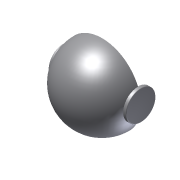
# Autodesk Inventor part: Head
Saved by Autodesk Inventor 2011 (Build 150239000, 239)
## iProperties
Created: 2011-04-09
Part Number: Head
Document SubType Name: Modeling
Designer: Milton
Density: 1 g/cm^3
Author: Milton
Autodesk Inventor part; units mm, degrees
sketch "Sketch1" plane through (0, 0, 0) normal (0, 0, 1) x (1, 0, 0)
  arc A0 (-59, 0) -> (59, 0) centre (0, 0) ccw
  arc A1 (-58, 0) -> (58, 0) centre (0, 0) ccw
  line L0 (-59, 0) -> (59, 0)
  dimension "d0" = 118
  dimension "d1" = 116
  constraints: 4 point on circle, 2 centre point, 2 coincident, 2 end point, 2 point on line
  measures "d0" diameter of A0
  measures "d1" diameter of A1
revolve "Revolution1" add sketch "Sketch1" angle 360 about axis through (-59, 0, 0) along (1, 0, 0) contours L0 A1 A0
ref_plane "Work Plane1" through (0, 0, 59) normal (0, 0, 1) x (1, 0, 0)
sketch "Sketch2" plane through (0, 0, 59) normal (0, 0, 1) x (1, 0, 0)
  circle A0 centre (0, 0) radius 59 projected
  line L0 (-59, 0) -> (59, 0)
  constraints: 2 end point, 2 point on circle, 1 horizontal
extrude "Extrusion1" cut sketch "Sketch2" against normal through all contours L0 A0 picked at (13.5288, 25.207)
ref_plane "Work Plane2" through (-59, 0, 0) normal (1, 0, 0) x (0, 1, 0)
sketch "Sketch3" plane through (-59, 0, 0) normal (1, 0, 0) x (0, 1, 0)
  circle A0 centre (0, 0) radius 22.5
  dimension "d5" = 45
  constraints: 1 centre point, 1 coincident
  measures "d5" diameter of A0
extrude "Extrusion2" add sketch "Sketch3" along normal blind 5
fillet "Fillet1" radius 1 1 edges at (-59, -22.5, 0)
ref_plane "Work Plane3" through (59, 0, 0) normal (1, 0, 0) x (0, 1, 0)
sketch "Sketch4" plane through (59, 0, 0) normal (1, 0, 0) x (0, 1, 0)
  circle A0 centre (0, 0) radius 22.5
  point P0 (0, 22.5)
  constraints: 1 coincident, 1 vertical alignment, 2 other
extrude "Extrusion3" add sketch "Sketch4" against normal blind 5
fillet "Fillet2" radius 1 1 edges at (59, -22.5, 0)
body "Solid1"
